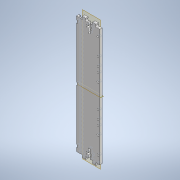
# Autodesk Inventor part: side_bottom
Saved by Autodesk Inventor 2020 (Build 240168000, 168)
## iProperties
Created: 2020-01-09
Part Number: side_bottom
Material: Generic
Document SubType Name: Modeling
Designer: erwin
Density: 1 g/cm^3
Appearance: Default
Author: erwin
Autodesk Inventor part; units mm, degrees
ref_plane "YZ Plane" through (0, 0, 0) normal (1, 0, 0) x (0, 1, 0)
ref_plane "XZ Plane" through (0, 0, 0) normal (0, 1, 0) x (-1, 0, 0)
ref_plane "XY Plane" through (0, 0, 0) normal (0, 0, 1) x (1, 0, 0)
ref_plane "Work Plane1" through (0, 0, 0) normal (0, 0, 1) x (1, 0, 0)
sketch "Sketch1" plane through (0, 0, 0) normal (0, 0, 1) x (1, 0, 0)
  line L0 (0, 0) -> (0, 170) projected
  line L1 (0, 170) -> (-24, 170) projected
  line L2 (-24, 0) -> (-24, 170) projected
  line L3 (0, 0) -> (-24, 0) projected
  line L4 (-27.6, 173.6) -> (3.6, 173.6)
  line L5 (3.6, 173.6) -> (3.6, -3.6)
  line L6 (3.6, -3.6) -> (-27.6, -3.6)
  line L7 (-27.6, -3.6) -> (-27.6, 173.6)
  line L8 (3.6, 10) -> (3.6, -1.8) projected
  line L9 (0, 10) -> (3.6, 10) projected
  line L10 (0, 0) -> (0, 10) projected
  line L11 (0, -1.8) -> (3.6, -1.8) projected
  line L12 (3.6, 131.2201) -> (3.6, 125.1799) projected
  line L13 (0, 125.1799) -> (0, 131.2201) projected
  line L14 (3.6, 131.2201) -> (3.6, 125.1799) projected
  line L15 (0, 125.1799) -> (0, 131.2201) projected
  line L16 (3.6, 131.2201) -> (3.6, 125.1799) projected
  line L17 (0, 125.1799) -> (0, 131.2201) projected
  line L18 (3.6, 131.2201) -> (3.6, 125.1799) projected
  line L19 (0, 125.1799) -> (0, 131.2201) projected
  line L20 (3.6, 170) -> (3.6, 160)
  line L21 (0, 170) -> (3.6, 170)
  line L22 (0, 160) -> (0, 170)
  line L23 (0, 160) -> (3.6, 160)
  line L24 (0, 125.1799) -> (3.6, 125.1799) projected
  line L25 (3.6, 131.2201) -> (0, 131.2201) projected
  line L26 (0, 125.1799) -> (3.6, 125.1799) projected
  line L27 (3.6, 131.2201) -> (0, 131.2201) projected
  line L28 (0, 125.1799) -> (3.6, 125.1799) projected
  line L29 (3.6, 131.2201) -> (0, 131.2201) projected
  line L30 (0, 125.1799) -> (3.6, 125.1799) projected
  line L31 (3.6, 131.2201) -> (0, 131.2201) projected
  point P0 (3.6, 46.8)
  point P1 (3.6, 36.8)
  point P2 (0, 46.8)
  point P3 (0, 36.8)
  point P4 (3.6, 66.8)
  point P5 (3.6, 56.8)
  point P6 (0, 66.8)
  point P7 (0, 56.8)
  point P8 (3.6, 113.2)
  point P9 (3.6, 103.2)
  point P10 (0, 113.2)
  point P11 (0, 103.2)
  point P12 (3.6, 133.2)
  point P13 (3.6, 123.2)
  point P14 (0, 133.2)
  point P15 (0, 123.2)
  dimension "d0" = 3.6
  constraints: 14 end point, 2 parallel, 5 other
  measures "d0" distance between parallel lines of L2 L7
extrude "Extrusion1" add sketch "Sketch1" along normal blind 3.6
sketch "Sketch2" plane through (0, 0, 3.6) normal (0, 0, 1) x (1, 0, 0)
  line L0 (3.6, -3.6) -> (3.6, 173.6) projected
  line L1 (3.6, 173.6) -> (-27.6, 173.6) projected
  line L2 (-27.6, 173.6) -> (-27.6, -3.6) projected
  line L3 (-27.6, -3.6) -> (3.6, -3.6) projected
  line L4 (-17, -3.6) -> (-7, -3.6)
  line L5 (-7, -3.6) -> (-7, 0)
  line L6 (-7, 0) -> (-17, 0)
  line L7 (-17, 0) -> (-17, -3.6)
  line L8 (-17, -3.6) -> (-22, -3.6)
  line L9 (-22, -3.6) -> (-22, 0)
  line L10 (-22, 0) -> (-17, 0)
  line L11 (-17, 0) -> (-17, -3.6)
  line L12 (-7, -3.6) -> (-2, -3.6)
  line L13 (-2, -3.6) -> (-2, 0)
  line L14 (-2, 0) -> (-7, 0)
  line L15 (-7, 0) -> (-7, -3.6)
  line L16 (-22, 0) -> (-27.6, 0)
  line L17 (-27.6, 0) -> (-27.6, -3.6)
  line L18 (-27.6, -3.6) -> (-22, -3.6)
  line L19 (-22, -3.6) -> (-22, 0)
  line L20 (-27.6, -3.6) -> (3.6, -3.6) projected
  line L21 (-2, 0) -> (3.6, 0)
  line L22 (3.6, 0) -> (3.6, -3.6)
  line L23 (3.6, -3.6) -> (-2, -3.6)
  line L24 (-2, -3.6) -> (-2, 0)
  line L25 (-13.5, -13) -> (-10.5, -13)
  line L26 (-10.5, -13) -> (-10.5, 13)
  line L27 (-10.5, 13) -> (-13.5, 13)
  line L28 (-13.5, 13) -> (-13.5, -13)
  line L29 (-13.5, -13) -> (-10.5, 13) construction
  line L30 (-10.5, -13) -> (-13.5, 13) construction
  line L31 (-16, 4) -> (-8, 4)
  line L32 (-8, 4) -> (-8, 7)
  line L33 (-8, 7) -> (-16, 7)
  line L34 (-16, 7) -> (-16, 4)
  line L35 (-16, 4) -> (-8, 7) construction
  line L36 (-8, 4) -> (-16, 7) construction
  line L37 (-12, 13) -> (-12, 0) construction
  point P0 (0, 0)
  point P1 (-12, 5.5)
  point P2 (-12, 5.5)
  point P3 (-13.5, 4)
  point P4 (-13.5, 0)
  point P5 (-10.5, 0)
  point P6 (-10.5, 4)
  point P7 (-10.5, 7)
  point P8 (-13.5, 7)
  dimension "d3" = 10
  dimension "d4" = 3.6
  dimension "d5" = 10.6
  dimension "d7" = 5
  dimension "d8" = 5
  dimension "d9" = 3
  dimension "d10" = 26
  dimension "d11" = 8
  dimension "d12" = 3
  dimension "d14" = 4
  constraints: 66 end point, 15 parallel, 7 horizontal, 7 midpoint, 7 perpendicular, 3 point on line
  measures "d3" distance of L6.end L5.end
  measures "d4" distance of L5.end L4.end
  measures "d5" distance between parallel lines of L2 L7
  measures "d7" distance of L9.end L10.end
  measures "d8" distance of L14.end L13.end
  measures "d9" distance of L27.end L26.end
  measures "d10" distance of L26.end L25.end
  measures "d11" distance of L33.end L32.end
  measures "d12" distance of L32.end L31.end
  measures "d14" distance between parallel lines of L6 L31
extrude "Extrusion2" cut sketch "Sketch2" against normal blind 3.6 contours L3 L13 L21 L0 | L3 L26 L6 L5 | L3 L28 L6 L26 | L16 L9 L3 L2 | L6 L28 L31 L26 | L3 L7 L6 L28 | L31 L28 L33 L26 | L26 L33 L32 L31 | L31 L34 L33 L28 | L33 L28 L27 L26
ref_plane "Work Plane2" through (-22, 85, 0) normal (0, -1, 0) x (1, 0, 0)
mirror "Mirror1" about plane through (-22, 85, 0) normal (0, -1, 0) of "Extrusion2"
sketch "Sketch3" plane through (-27.6, 170, 3.6) normal (0, 1, 0) x (1, 0, 0)
  line L0 (27.6, 3.6) -> (27.6, 73.6) projected
  line L1 (27.6, 73.6) -> (3.6, 73.6) projected
  line L2 (3.6, 3.6) -> (3.6, 73.6) projected
  line L3 (27.6, 3.6) -> (3.6, 3.6) projected
  line L4 (5.6, 0) -> (0, 0) projected
  line L5 (5.6, 0) -> (5.6, 3.6) projected
  line L6 (0, 3.6) -> (5.6, 3.6) projected
  line L7 (0, 0) -> (0, 3.6) projected
  line L8 (0, 3.6) -> (0, 0) projected
  line L9 (3.6, 3.6) -> (0, 3.6)
  line L10 (0, 3.6) -> (0, 1.8)
  line L11 (0, 1.8) -> (3.6, 1.8)
  line L12 (3.6, 1.8) -> (3.6, 3.6)
  line L13 (0, 0) -> (-2.4, 0)
  line L14 (-2.4, 0) -> (-2.4, 3.6)
  line L15 (-2.4, 3.6) -> (0, 3.6)
  line L16 (0, 3.6) -> (0, 0)
  dimension "d17" = 2.4
  constraints: 16 end point, 4 parallel, 2 horizontal, 2 perpendicular, 1 midpoint, 1 point on line
  measures "d17" distance of L14.end L15.end
extrude "Extrusion3" add sketch "Sketch3" against normal up to surface (170 mm away) contours L7 L13 L14 L15
sketch "Sketch4" plane through (-22, 170, 3.6) normal (0, 1, 0) x (1, 0, 0)
  line L0 (-8, 0) -> (0, 0) projected
  line L1 (0, 0) -> (0, 3.6) projected
  line L2 (-8, 3.6) -> (0, 3.6) projected
  line L3 (-8, 3.6) -> (-8, 0) projected
  line L4 (22, 3.6) -> (22, 73.6) projected
  line L5 (22, 73.6) -> (-2, 73.6) projected
  line L6 (-2, 3.6) -> (-2, 73.6) projected
  line L7 (22, 3.6) -> (-2, 3.6) projected
  line L8 (-2, 3.6) -> (-6, 3.6)
  line L9 (-6, 3.6) -> (-6, 1.8)
  line L10 (-6, 1.8) -> (-2, 1.8)
  line L11 (-2, 1.8) -> (-2, 3.6)
  point P0 (-6, 3.6)
  dimension "d20" = 4
  dimension "d21" = 1.8
  constraints: 8 end point, 2 parallel, 1 horizontal, 1 perpendicular
  measures "d20" distance of L10.end L9.end
  measures "d21" distance of L8.end L9.end
extrude "Extrusion4" cut sketch "Sketch4" against normal through all contours L2 L11 L10 L9
sketch "Sketch5" plane through (0, 0, 0) normal (0, 0, -1) x (-1, 0, 0)
  line L0 (28, 170) -> (28, 0) projected
  line L1 (28, 0) -> (30, 0) projected
  line L2 (30, 170) -> (30, 0) projected
  line L3 (30, 170) -> (28, 170) projected
  line L4 (29, 83) -> (31, 83)
  line L5 (31, 83) -> (31, 87)
  line L6 (31, 87) -> (29, 87)
  line L7 (29, 87) -> (29, 83)
  line L8 (30, 170) -> (30, 0) projected
  line L9 (29, 83) -> (31, 87) construction
  line L10 (31, 83) -> (29, 87) construction
  line L11 (29, 165) -> (31, 165)
  line L12 (31, 165) -> (31, 161)
  line L13 (31, 161) -> (29, 161)
  line L14 (29, 161) -> (29, 165)
  line L15 (30, 170) -> (30, 0) projected
  line L16 (29, 165) -> (31, 161) construction
  line L17 (31, 165) -> (29, 161) construction
  line L18 (30, 85) -> (40.6182, 85) construction
  line L19 (30, 0) -> (28, 0)
  line L20 (29, 5) -> (31, 5)
  line L21 (31, 5) -> (31, 9)
  line L22 (31, 9) -> (29, 9)
  line L23 (29, 9) -> (29, 5)
  line L24 (29, 5) -> (31, 9) construction
  line L25 (31, 5) -> (29, 9) construction
  point P0 (0, 0)
  point P1 (30, 163)
  point P2 (30, 7)
  point P3 (30, 5)
  point P4 (30, 9)
  point P5 (30, 83)
  point P6 (30, 87)
  point P7 (30, 161)
  point P8 (30, 165)
  dimension "d24" = 2
  dimension "d25" = 4
  dimension "d26" = 4
  dimension "d27" = 5
  constraints: 40 end point, 7 midpoint, 5 symmetric about line, 4 parallel, 3 horizontal, 2 perpendicular, 1 point on line
  measures "d24" distance of L6.end L5.end
  measures "d25" distance of L5.end L4.end
  measures "d26" distance of L11.end L12.end
  measures "d27" vertical distance of L2.start L11.end
extrude "Extrusion5" cut sketch "Sketch5" against normal through all contours L2 L13 L14 L11 | L20 L23 L22 L2 | L2 L4 L7 L6
sketch "Sketch6" plane through (0, 0, 3.6) normal (0, 0, 1) x (1, 0, 0)
  line L0 (-29, 5) -> (-30, 5) projected
  line L1 (-30, 5) -> (-30, 0) projected
  line L2 (-30, 0) -> (-22, 0) projected
  line L3 (-22, 0) -> (-22, -3.6) projected
  line L4 (-22, -3.6) -> (-17, -3.6) projected
  line L5 (-17, -3.6) -> (-17, 0) projected
  line L6 (-17, 0) -> (-13.5, 0) projected
  line L7 (-13.5, 0) -> (-13.5, 4) projected
  line L8 (-13.5, 4) -> (-16, 4) projected
  line L9 (-16, 4) -> (-16, 7) projected
  line L10 (-16, 7) -> (-13.5, 7) projected
  line L11 (-13.5, 7) -> (-13.5, 13) projected
  line L12 (-13.5, 13) -> (-10.5, 13) projected
  line L13 (-10.5, 13) -> (-10.5, 7) projected
  line L14 (-10.5, 7) -> (-8, 7) projected
  line L15 (-8, 7) -> (-8, 4) projected
  line L16 (-8, 4) -> (-10.5, 4) projected
  line L17 (-10.5, 4) -> (-10.5, 0) projected
  line L18 (-10.5, 0) -> (-7, 0) projected
  line L19 (-7, 0) -> (-7, -3.6) projected
  line L20 (-7, -3.6) -> (-2, -3.6) projected
  line L21 (-2, -3.6) -> (-2, 0) projected
  line L22 (-2, 0) -> (3.6, 0) projected
  line L23 (3.6, 0) -> (3.6, 170) projected
  line L24 (3.6, 170) -> (-2, 170) projected
  line L25 (-2, 170) -> (-2, 173.6) projected
  line L26 (-2, 173.6) -> (-7, 173.6) projected
  line L27 (-7, 173.6) -> (-7, 170) projected
  line L28 (-7, 170) -> (-10.5, 170) projected
  line L29 (-10.5, 170) -> (-10.5, 166) projected
  line L30 (-10.5, 166) -> (-8, 166) projected
  line L31 (-8, 166) -> (-8, 163) projected
  line L32 (-8, 163) -> (-10.5, 163) projected
  line L33 (-10.5, 163) -> (-10.5, 157) projected
  line L34 (-10.5, 157) -> (-13.5, 157) projected
  line L35 (-13.5, 157) -> (-13.5, 163) projected
  line L36 (-13.5, 163) -> (-16, 163) projected
  line L37 (-16, 163) -> (-16, 166) projected
  line L38 (-16, 166) -> (-13.5, 166) projected
  line L39 (-13.5, 166) -> (-13.5, 170) projected
  line L40 (-13.5, 170) -> (-17, 170) projected
  line L41 (-17, 170) -> (-17, 173.6) projected
  line L42 (-17, 173.6) -> (-22, 173.6) projected
  line L43 (-22, 173.6) -> (-22, 170) projected
  line L44 (-30, 170) -> (-22, 170) projected
  line L45 (-30, 170) -> (-30, 165) projected
  line L46 (-30, 165) -> (-29, 165) projected
  line L47 (-29, 165) -> (-29, 161) projected
  line L48 (-29, 161) -> (-30, 161) projected
  line L49 (-30, 161) -> (-30, 87) projected
  line L50 (-30, 87) -> (-29, 87) projected
  line L51 (-29, 87) -> (-29, 83) projected
  line L52 (-29, 83) -> (-30, 83) projected
  line L53 (-30, 83) -> (-30, 9) projected
  line L54 (-30, 9) -> (-29, 9) projected
  line L55 (-29, 9) -> (-29, 5) projected
  circle A0 centre (-28.3256, -9.1766) radius 1.4 construction
  line L56 (-29.3156, -10.1665) -> (-27.3357, -10.1665) construction
  line L57 (-27.3357, -10.1665) -> (-27.3357, -8.1866) construction
  line L58 (-27.3357, -8.1866) -> (-29.3156, -8.1866) construction
  line L59 (-29.3156, -8.1866) -> (-29.3156, -10.1665) construction
  line L60 (-29.3156, -10.1665) -> (-27.3357, -8.1866) construction
  line L61 (-27.3357, -10.1665) -> (-29.3156, -8.1866) construction
  line L62 (-21.0101, 0.9899) -> (-22.9899, 0.9899)
  line L63 (-22.9899, 0.9899) -> (-22.9899, -0.9899)
  line L64 (-22.9899, -0.9899) -> (-21.0101, -0.9899)
  line L65 (-21.0101, -0.9899) -> (-21.0101, 0.9899)
  line L66 (-22, 0) -> (-24, 0) projected
  line L67 (-21.0101, 0.9899) -> (-22.9899, -0.9899) construction
  line L68 (-22.9899, 0.9899) -> (-21.0101, -0.9899) construction
  line L69 (-17.9899, 0.9899) -> (-16.0101, 0.9899)
  line L70 (-16.0101, 0.9899) -> (-16.0101, -0.9899)
  line L71 (-16.0101, -0.9899) -> (-17.9899, -0.9899)
  line L72 (-17.9899, -0.9899) -> (-17.9899, 0.9899)
  line L73 (-17, 0) -> (-17, -3.6) projected
  line L74 (-17.9899, 0.9899) -> (-16.0101, -0.9899) construction
  line L75 (-16.0101, 0.9899) -> (-17.9899, -0.9899) construction
  line L76 (-6.0101, 0.9899) -> (-7.9899, 0.9899)
  line L77 (-7.9899, 0.9899) -> (-7.9899, -0.9899)
  line L78 (-7.9899, -0.9899) -> (-6.0101, -0.9899)
  line L79 (-6.0101, -0.9899) -> (-6.0101, 0.9899)
  line L80 (-6.0101, 0.9899) -> (-7.9899, -0.9899) construction
  line L81 (-7.9899, 0.9899) -> (-6.0101, -0.9899) construction
  line L82 (-2.9899, 0.9899) -> (-1.0101, 0.9899)
  line L83 (-1.0101, 0.9899) -> (-1.0101, -0.9899)
  line L84 (-1.0101, -0.9899) -> (-2.9899, -0.9899)
  line L85 (-2.9899, -0.9899) -> (-2.9899, 0.9899)
  line L86 (3.6, 0) -> (-2, 0) projected
  line L87 (-2.9899, 0.9899) -> (-1.0101, -0.9899) construction
  line L88 (-1.0101, 0.9899) -> (-2.9899, -0.9899) construction
  line L89 (-0.9899, 9.0101) -> (0.9899, 9.0101)
  line L90 (0.9899, 9.0101) -> (0.9899, 10.9899)
  line L91 (0.9899, 10.9899) -> (-0.9899, 10.9899)
  line L92 (-0.9899, 10.9899) -> (-0.9899, 9.0101)
  line L93 (-0.9899, 9.0101) -> (0.9899, 10.9899) construction
  line L94 (0.9899, 9.0101) -> (-0.9899, 10.9899) construction
  line L95 (-0.9899, 37.7899) -> (0.9899, 37.7899)
  line L96 (0.9899, 37.7899) -> (0.9899, 35.8101)
  line L97 (0.9899, 35.8101) -> (-0.9899, 35.8101)
  line L98 (-0.9899, 35.8101) -> (-0.9899, 37.7899)
  line L99 (-0.9899, 37.7899) -> (0.9899, 35.8101) construction
  line L100 (0.9899, 37.7899) -> (-0.9899, 35.8101) construction
  line L101 (-0.9899, 65.8101) -> (0.9899, 65.8101)
  line L102 (0.9899, 65.8101) -> (0.9899, 67.7899)
  line L103 (0.9899, 67.7899) -> (-0.9899, 67.7899)
  line L104 (-0.9899, 67.7899) -> (-0.9899, 65.8101)
  line L105 (0, 66.8) -> (0, 103.2) projected
  line L106 (-0.9899, 65.8101) -> (0.9899, 67.7899) construction
  line L107 (0.9899, 65.8101) -> (-0.9899, 67.7899) construction
  line L108 (-0.9899, 104.1899) -> (0.9899, 104.1899)
  line L109 (0.9899, 104.1899) -> (0.9899, 102.2101)
  line L110 (0.9899, 102.2101) -> (-0.9899, 102.2101)
  line L111 (-0.9899, 102.2101) -> (-0.9899, 104.1899)
  line L112 (-0.9899, 104.1899) -> (0.9899, 102.2101) construction
  line L113 (0.9899, 104.1899) -> (-0.9899, 102.2101) construction
  line L114 (-0.9899, 112.2101) -> (0.9899, 112.2101)
  line L115 (0.9899, 112.2101) -> (0.9899, 114.1899)
  line L116 (0.9899, 114.1899) -> (-0.9899, 114.1899)
  line L117 (-0.9899, 114.1899) -> (-0.9899, 112.2101)
  line L118 (3.6, 113.2) -> (0, 113.2) projected
  line L119 (-0.9899, 112.2101) -> (0.9899, 114.1899) construction
  line L120 (0.9899, 112.2101) -> (-0.9899, 114.1899) construction
  line L121 (-0.9899, 124.1899) -> (0.9899, 124.1899)
  line L122 (0.9899, 124.1899) -> (0.9899, 122.2101)
  line L123 (0.9899, 122.2101) -> (-0.9899, 122.2101)
  line L124 (-0.9899, 122.2101) -> (-0.9899, 124.1899)
  line L125 (0, 123.2) -> (3.6, 123.2) projected
  line L126 (-0.9899, 124.1899) -> (0.9899, 122.2101) construction
  line L127 (0.9899, 124.1899) -> (-0.9899, 122.2101) construction
  line L128 (-0.9899, 132.2101) -> (0.9899, 132.2101)
  line L129 (0.9899, 132.2101) -> (0.9899, 134.1899)
  line L130 (0.9899, 134.1899) -> (-0.9899, 134.1899)
  line L131 (-0.9899, 134.1899) -> (-0.9899, 132.2101)
  line L132 (3.6, 133.2) -> (0, 133.2) projected
  line L133 (-0.9899, 132.2101) -> (0.9899, 134.1899) construction
  line L134 (0.9899, 132.2101) -> (-0.9899, 134.1899) construction
  line L135 (-0.9899, 160.9899) -> (0.9899, 160.9899)
  line L136 (0.9899, 160.9899) -> (0.9899, 159.0101)
  line L137 (0.9899, 159.0101) -> (-0.9899, 159.0101)
  line L138 (-0.9899, 159.0101) -> (-0.9899, 160.9899)
  line L139 (0, 133.2) -> (0, 160) projected
  line L140 (-0.9899, 160.9899) -> (0.9899, 159.0101) construction
  line L141 (0.9899, 160.9899) -> (-0.9899, 159.0101) construction
  line L142 (-7.9899, 170.9899) -> (-6.0101, 170.9899)
  line L143 (-6.0101, 170.9899) -> (-6.0101, 169.0101)
  line L144 (-6.0101, 169.0101) -> (-7.9899, 169.0101)
  line L145 (-7.9899, 169.0101) -> (-7.9899, 170.9899)
  line L146 (-7.9899, 170.9899) -> (-6.0101, 169.0101) construction
  line L147 (-6.0101, 170.9899) -> (-7.9899, 169.0101) construction
  line L148 (-1.1868, 170.8132) -> (-2.8132, 170.8132)
  line L149 (-2.8132, 170.8132) -> (-2.8132, 169.1868)
  line L150 (-2.8132, 169.1868) -> (-1.1868, 169.1868)
  line L151 (-1.1868, 169.1868) -> (-1.1868, 170.8132)
  line L152 (-1.1868, 170.8132) -> (-2.8132, 169.1868) construction
  line L153 (-2.8132, 170.8132) -> (-1.1868, 169.1868) construction
  line L154 (-17.8132, 170.8132) -> (-16.1868, 170.8132)
  line L155 (-16.1868, 170.8132) -> (-16.1868, 169.1868)
  line L156 (-16.1868, 169.1868) -> (-17.8132, 169.1868)
  line L157 (-17.8132, 169.1868) -> (-17.8132, 170.8132)
  line L158 (-17.8132, 170.8132) -> (-16.1868, 169.1868) construction
  line L159 (-16.1868, 170.8132) -> (-17.8132, 169.1868) construction
  line L160 (-22.8132, 170.8132) -> (-21.1868, 170.8132)
  line L161 (-21.1868, 170.8132) -> (-21.1868, 169.1868)
  line L162 (-21.1868, 169.1868) -> (-22.8132, 169.1868)
  line L163 (-22.8132, 169.1868) -> (-22.8132, 170.8132)
  line L164 (-22.8132, 170.8132) -> (-21.1868, 169.1868) construction
  line L165 (-21.1868, 170.8132) -> (-22.8132, 169.1868) construction
  line L166 (-0.9899, 57.7899) -> (0.9899, 57.7899)
  line L167 (0.9899, 57.7899) -> (0.9899, 55.8101)
  line L168 (0.9899, 55.8101) -> (-0.9899, 55.8101)
  line L169 (-0.9899, 55.8101) -> (-0.9899, 57.7899)
  line L170 (-0.9899, 57.7899) -> (0.9899, 55.8101) construction
  line L171 (0.9899, 57.7899) -> (-0.9899, 55.8101) construction
  line L172 (-0.9899, 45.8101) -> (0.9899, 45.8101)
  line L173 (0.9899, 45.8101) -> (0.9899, 47.7899)
  line L174 (0.9899, 47.7899) -> (-0.9899, 47.7899)
  line L175 (-0.9899, 47.7899) -> (-0.9899, 45.8101)
  line L176 (-0.9899, 45.8101) -> (0.9899, 47.7899) construction
  line L177 (0.9899, 45.8101) -> (-0.9899, 47.7899) construction
  point P0 (0, 0)
  point P1 (0, 10)
  point P2 (0, 36.8)
  point P3 (0, 46.8)
  point P4 (0, 56.8)
  point P5 (0.8132, 159.1868)
  point P6 (0.8132, 102.3868)
  point P7 (0.8132, 35.9868)
  dimension "d30" = 2.8
  dimension "d32" = 1.9799
  dimension "d33" = 1.9799
  constraints: 228 end point, 38 midpoint, 38 parallel, 19 equal length, 19 horizontal, 19 perpendicular, 16 coincident, 13 point on line, 3 other
  measures "d32" distance of L57.end L58.end
  measures "d33" distance of L63.end L64.end
hole "Hole1" at (-28.3256, -9.1766, 3.6) at (-22.8132, 170.8132, 3.6) at (-16.1868, 170.8132, 3.6) at (-7.9899, 170.9899, 3.6) at (-1.1868, 170.8132, 3.6) at (0.8132, 159.1868, 3.6) at (0.9899, 134.1899, 3.6) at (0.9899, 122.2101, 3.6) at (0.9899, 114.1899, 3.6) at (0.8132, 102.3868, 3.6) at (0.9899, 67.7899, 3.6) at (0.9899, 55.8101, 3.6) at (0.9899, 47.7899, 3.6) at (0.8132, 35.9868, 3.6) at (0.9899, 10.9899, 3.6) at (-1.0101, -0.9899, 3.6) at (-7.9899, -0.9899, 3.6) at (-16.0101, -0.9899, 3.6) at (-22.9899, -0.9899, 3.6) direction (0, 0, -1) diameter 2.8 end through all
equation "\"d0\" = wood_thickness"
equation "\"d1\" = wood_thickness"
equation "\"d3\" = tabs_width"
equation "\"d4\" = wood_thickness"
equation "\"d7\" = 0.5 * tabs_width"
equation "\"d8\" = 0.5 * tabs_width"
equation "\"d9\" = screw_diameter"
equation "\"d10\" = 2 * screw_depth"
equation "\"d11\" = screw_nut_width"
equation "\"d12\" = screw_nut_thickness"
equation "\"d20\" = wood_thickness + extra_for_sliding_cover"
equation "\"d21\" = deep_for_sliding_cover"
equation "\"d26\" = d25"
equation "\"d30\" = bit_diameter"
equation "\"d33\" = d32"
equation "\"d34\" = bit_diameter"
equation "\"wood_thickness\" = 3.6"
equation "\"tabs_width\" = 10"
equation "\"screw_diameter\" = 3"
equation "\"screw_depth\" = 13"
equation "\"screw_nut_width\" = 8"
equation "\"screw_nut_thickness\" = 3"
equation "\"extra_for_sliding_cover\" = 0.4"
equation "\"deep_for_sliding_cover\" = 1.8"
equation "\"bit_diameter\" = 2.8"
body "Solid1"
